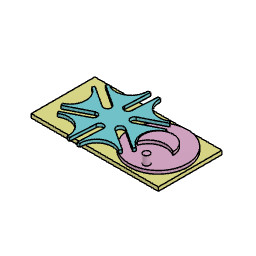
6 Slotted Geneva Mechanism v4 (Autodesk Fusion 360 design; units mm, degrees)
Autodesk Fusion 360 part; units mm, degrees
note: some values were not read from the file. Chosen so that the rebuilt part matches the saved one: which face or edge a step refers to. Set by a fixed rule: which sketch regions a step uses.
sketch "Holder" plane through (0, 0, 0) normal (0, 0, 1) x (1, 0, 0) in component "Holder"
  line L0 (100, -50) -> (-100, -50)
  line L1 (-100, -50) -> (-100, 50)
  line L2 (-100, 50) -> (100, 50)
  line L3 (100, 50) -> (100, -50)
  line L4 (100, -50) -> (-100, 50) construction
  line L5 (-100, -50) -> (100, 50) construction
  constraint horizontal L0
  constraint perpendicular L0 L1
  constraint parallel L0 L2
  constraint parallel L1 L3
  constraint coincident L4 origin
  constraint coincident L5 origin
extrude "Extrude1" add sketch "Holder" along normal blind 6 makes body 1 in component "Holder"
sketch "crank" plane through (0, 0, 6) normal (0, 0, 1) x (-1, 0, 0) in component "Crank"
  line L0 (-100, -50) -> (100, -50)
  line L1 (100, -50) -> (100, 50)
  line L2 (100, 50) -> (-100, 50)
  line L3 (-100, 50) -> (-100, -50)
  line L4 (100, 0) -> (-100, 0) construction
  line L5 (0, -50) -> (0, 50) construction
  line L6 (0, 0) -> (-100, 0) construction
  line L7 (-50, 0) -> (-50, -50) construction
  circle A0 centre (-50, 0) radius 46.0977
  constraint midpoint L1 L4.start
  constraint midpoint L3 L4.end
  constraint midpoint L0 L5.start
  constraint midpoint L2 L5.end
  constraint coincident L6.start origin
  constraint midpoint L6 L7.start
  constraint coincident L0 L7.end
  constraint perpendicular L0 L7
  constraint coincident L7.start A0.centre
extrude "Extrude1'" add sketch "crank" along normal blind 5 separate body contours A0 makes body 2 in component "Crank"
sketch "rotating point" plane through (0, 0, 6) normal (0, 0, -1) x (1, 0, 0) in component "Crank"
  circle A0 centre (50, 0) radius 46.0977
  circle A1 centre (50, 0) radius 5
  dimension "d7" = 10
  constraint concentric A0 A1
  measures "d7" diameter of A1
sketch "crank hole" plane through (0, 0, 0) normal (0, 0, -1) x (1, 0, 0) in component "Holder"
  line L0 (-100, -50) -> (100, -50)
  line L1 (100, -50) -> (100, 50)
  line L2 (100, 50) -> (-100, 50)
  line L3 (-100, 50) -> (-100, -50)
  circle A0 centre (50, 0) radius 5
  dimension "d8" = 10
  measures "d8" diameter of A0
extrude "Extrude2" cut sketch "crank hole" against normal blind 21 contours A0 bodies 1 in component "Holder"
extrude "Extrude2'" add sketch "rotating point" along normal blind 6 contours A1 bodies 2 in component "Crank"
move_face "OffsetFaces1" offset -0.5 1 faces at (54.9938, 0.2492, 2) on bodies 2 in component "Crank"
sketch "middle circle" plane through (0, 0, 11) normal (0, 0, 1) x (-1, 0, 0) in component "Crank"
  circle A0 centre (-50, 0) radius 46.0977
  circle A1 centre (-50, 0) radius 24.5
  circle A2 centre (-74.4998, -0.0916) radius 27.5
  dimension "d14" = 49
  dimension "d15" = 55
  constraint concentric A0 A1
  constraint coincident A1 A2.centre
  measures "d14" diameter of A1
  measures "d15" diameter of A2
extrude "Extrude3" add sketch "middle circle" along normal blind 5 contours A1 A2 picked at (-40.002, 2.3523) bodies 2 in component "Crank"
sketch "contact rod" plane through (0, 0, 11) normal (0, 0, 1) x (-1, 0, 0) in component "Crank"
  arc A0 (-58.9812, -22.7945) -> (-59.1513, 22.7267) centre (-74.4998, -0.0916) ccw
  arc A1 (-58.9812, -22.7945) -> (-59.1513, 22.7267) centre (-50, 0) ccw
  circle A2 centre (-50, 0) radius 46.0977
  line L0 (-50, 0) -> (-95, 0) construction
  line L1 (-95, 0) -> (-72.5, 0) construction
  circle A3 centre (-83.75, 0) radius 5
  dimension "d18" = 10
  constraint coincident A1.centre A2.centre
  constraint horizontal L0
  constraint midpoint L0 L1.end
  constraint midpoint L1 A3.centre
  measures "d18" diameter of A3
extrude "Extrude4" add sketch "contact rod" against normal blind 5 contours A3 bodies 2 in component "Crank"
sketch "star " plane through (0, 0, 6) normal (0, 0, 1) x (-1, 0, 0) in component "Rotating star"
  circle A0 centre (-50, 0) radius 5
  line L0 (-100, -50) -> (100, -50)
  line L1 (100, -50) -> (100, 50)
  line L2 (100, 50) -> (-100, 50)
  line L3 (-100, 50) -> (-100, -50)
  line L4 (0, 0) -> (2.6271, 0)
  line L5 (2.6271, 0) -> (100, 0) construction
  line L6 (0, 0) -> (51.3135, 0) construction
  circle A1 centre (20, 0) radius 63.198
  circle A2 centre (-50, 0) radius 25
  dimension "d21" = 50
  constraint coincident L4.start L6.start
  constraint horizontal L4
  constraint midpoint L1 L5.end
  constraint perpendicular L1 L5
  constraint midpoint L5 L6.end
  constraint coincident L5 A1.centre
  constraint concentric A0 A2
  measures "d21" diameter of A2
extrude "Extrude1''" add sketch "star " along normal blind 10 separate body contours L0 L2 A1 A2 | L0 A1 | L2 A1 makes body 3 in component "Rotating star"
move_face "OffsetFaces1'" offset -5 1 faces at (-28.1206, -36.1937, 6) on bodies 3 in component "Rotating star"
pattern_circular "C-Pattern1" count 6 over 360 about axis through (-20, 0, 16) along (0, 0, 1) of 2 faces at (38.0291, -21.9476, 14.3333) (27.6641, 11.2297, 14.3333) on bodies 3 in component "Rotating star"
sketch "Hole" plane through (0, 0, 16) normal (0, 0, 1) x (-1, 0, 0) in component "Rotating star"
  arc A0 (-29.0014, 39.9104) -> (9.9373, 62.3917) centre (-15, 60.6218) ccw
  arc A1 (-29.0014, 39.9104) -> (-39.0642, 22.4813) centre (20, 0) ccw
  arc A2 (-39.0642, -22.4813) -> (-39.0642, 22.4813) centre (-50, 0) ccw
  arc A3 (-39.0642, -22.4813) -> (-29.0014, -39.9104) centre (20, 0) ccw
  arc A4 (9.9373, -62.3917) -> (-29.0014, -39.9104) centre (-15, -60.6218) ccw
  arc A5 (9.9373, -62.3917) -> (30.0627, -62.3917) centre (20, 0) ccw
  arc A6 (69.0014, -39.9104) -> (30.0627, -62.3917) centre (55, -60.6218) ccw
  arc A7 (69.0014, -39.9104) -> (79.0642, -22.4813) centre (20, 0) ccw
  arc A8 (79.0642, 22.4813) -> (79.0642, -22.4813) centre (90, 0) ccw
  arc A9 (79.0642, 22.4813) -> (69.0014, 39.9104) centre (20, 0) ccw
  arc A10 (30.0627, 62.3917) -> (69.0014, 39.9104) centre (55, 60.6218) ccw
  arc A11 (30.0627, 62.3917) -> (9.9373, 62.3917) centre (20, 0) ccw
  line L0 (25, 0) -> (-34.731, -31.599) construction
  line L1 (-2.3358, -7.6734) -> (-37.5367, -26.2954)
  arc A12 (-37.5367, -26.2954) -> (-31.9253, -36.9026) centre (-34.731, -31.599) ccw
  line L2 (-31.9253, -36.9026) -> (3.2756, -18.2805)
  arc A13 (3.2756, -18.2805) -> (-2.3358, -7.6734) centre (0.4699, -12.977) ccw
  line L3 (0.4699, -12.977) -> (-34.731, -31.599) construction
  dimension "d27" = 12
  constraint midpoint A3 L0.end
  constraint tangent L1 A12
  constraint tangent A12 L2
  constraint parallel L1 L2
  constraint tangent L2 A13
  constraint tangent L1 A13
  constraint coincident L0.end A12.centre
  constraint parallel L0 L3
  measures "d27" distance of L1 L2
extrude "Extrude2''" cut sketch "Hole" against normal blind 20 contours A3 L1 L2 A13 bodies 3 in component "Rotating star"
pattern_circular "C-Pattern2" count 6 over 360 about axis through (-20, 0, 16) along (0, 0, 1) of "Extrude2''" in component "Rotating star"
sketch "support " plane through (0, 0, 11) normal (0, 0, -1) x (1, 0, 0) in component "Rotating star"
  line L0 (-2.1867, 15.5067) -> (31.4876, 36.6471)
  arc A0 (31.4876, 36.6471) -> (29.0014, 39.9104) centre (-20, 0) ccw
  arc A1 (-9.9373, 62.3917) -> (29.0014, 39.9104) centre (15, 60.6218) ccw
  arc A2 (-9.9373, 62.3917) -> (-13.9853, 62.9111) centre (-20, 0) ccw
  line L1 (-13.9853, 62.9111) -> (-12.5308, 23.6241)
  arc A3 (-24.5226, 23.1801) -> (-12.5308, 23.6241) centre (-18.5267, 23.4021) ccw
  line L2 (-24.5226, 23.1801) -> (-25.9936, 62.9131)
  arc A4 (-25.9936, 62.9131) -> (-30.0627, 62.3917) centre (-20, 0) ccw
  arc A5 (-69.0014, 39.9104) -> (-30.0627, 62.3917) centre (-55, 60.6218) ccw
  arc A6 (-69.0014, 39.9104) -> (-71.4752, 36.6645) centre (-20, 0) ccw
  line L3 (-71.4752, 36.6645) -> (-36.7244, 18.2805)
  arc A7 (-42.3358, 7.6734) -> (-36.7244, 18.2805) centre (-39.5301, 12.977) ccw
  line L4 (-42.3358, 7.6734) -> (-77.4811, 26.266)
  arc A8 (-77.4811, 26.266) -> (-79.0642, 22.4813) centre (-20, 0) ccw
  arc A9 (-79.0642, -22.4813) -> (-79.0642, 22.4813) centre (-90, 0) ccw
  arc A10 (-79.0642, -22.4813) -> (-77.49, -26.2466) centre (-20, 0) ccw
  line L5 (-77.49, -26.2466) -> (-44.1936, -5.3435)
  arc A11 (-37.8133, -15.5067) -> (-44.1936, -5.3435) centre (-41.0034, -10.4251) ccw
  line L6 (-37.8133, -15.5067) -> (-71.4876, -36.6471)
  arc A12 (-71.4876, -36.6471) -> (-69.0014, -39.9104) centre (-20, 0) ccw
  arc A13 (-30.0627, -62.3917) -> (-69.0014, -39.9104) centre (-55, -60.6218) ccw
  arc A14 (-30.0627, -62.3917) -> (-26.0147, -62.9111) centre (-20, 0) ccw
  line L7 (-26.0147, -62.9111) -> (-27.4692, -23.6241)
  arc A15 (-15.4774, -23.1801) -> (-27.4692, -23.6241) centre (-21.4733, -23.4021) ccw
  line L8 (-15.4774, -23.1801) -> (-14.0064, -62.9131)
  arc A16 (-14.0064, -62.9131) -> (-9.9373, -62.3917) centre (-20, 0) ccw
  arc A17 (29.0014, -39.9104) -> (-9.9373, -62.3917) centre (15, -60.6218) ccw
  arc A18 (29.0014, -39.9104) -> (31.4752, -36.6645) centre (-20, 0) ccw
  line L9 (31.4752, -36.6645) -> (-3.2756, -18.2805)
  arc A19 (2.3358, -7.6734) -> (-3.2756, -18.2805) centre (-0.4699, -12.977) ccw
  line L10 (2.3358, -7.6734) -> (37.4811, -26.266)
  arc A20 (37.4811, -26.266) -> (39.0642, -22.4813) centre (-20, 0) ccw
  arc A21 (39.0642, 22.4813) -> (39.0642, -22.4813) centre (50, 0) ccw
  arc A22 (39.0642, 22.4813) -> (37.49, 26.2466) centre (-20, 0) ccw
  line L11 (37.49, 26.2466) -> (4.1936, 5.3435)
  arc A23 (-2.1867, 15.5067) -> (4.1936, 5.3435) centre (1.0034, 10.4251) ccw
  circle A24 centre (-20, 0) radius 5
  dimension "d32" = 10
  constraint concentric A0 A24
  measures "d32" diameter of A24
sketch "star hole" plane through (0, 0, 0) normal (0, 0, -1) x (1, 0, 0) in component "Holder"
  circle A0 centre (50, 0) radius 5
  line L0 (-100, -50) -> (100, -50)
  line L1 (100, -50) -> (100, 50)
  line L2 (100, 50) -> (-100, 50)
  line L3 (-100, 50) -> (-100, -50)
  circle A1 centre (-20, 0) radius 5.5
  dimension "d33" = 11
  measures "d33" diameter of A1
extrude "Extrude3'" cut sketch "star hole" against normal blind 50 contours A1 bodies 1 in component "Holder"
extrude "Extrude3''" add sketch "support " along normal blind 11 contours A24 bodies 3 in component "Rotating star"
move_face "OffsetFaces2" offset -1 1 faces at (40.0739, -22.3992, 14.3333) on bodies 2 in component "Crank"
sketch "crank for the contact rod" plane through (67.101, 46.9846, 11) normal (0, 0, 1) x (0.34202, 0.939693, 0)
  arc A0 (-26.5, 0.0354) -> (-67.9116, -15.2127) centre (-41.5345, -22.991) ccw
  arc A1 (-26.5, 0.0354) -> (-67.9116, -15.2127) centre (-50, 0) ccw
  circle A2 centre (-50, 0) radius 46.0977
sketch "contact rod (2)" plane through (67.101, 46.9846, 11) normal (0, 0, 1) x (0.34202, 0.939693, 0)
  line L0 (-73.8686, 65.8531) -> (-50, 0) construction
  line L1 (-50, 0) -> (-27.4519, 26.7987) construction
  line L2 (-27.4519, 26.7987) -> (-73.8686, 65.8531) construction
  circle A0 centre (-27.4519, 26.7987) radius 5
  dimension "d50" = 30
  dimension "d51" = 60
  dimension "d52" = 10
  constraint coincident L1.end L2.start
  measures "d50" angle of L0 L2
  measures "d51" angle of L0 L1
  measures "d52" diameter of A0
extrude "Extrude5" add sketch "contact rod (2)" along normal blind 14 sketch seen with x (-0.422618, -0.906308, 0) y (0.906308, -0.422618, 0) z (0, 0, 1) at (71.1309, 45.3154, 0) bodies 2 in component "Crank"
component "Holder" placed x (1, 0, 0) y (0, 1, 0) z (0, 0, 1) at (0, 0, 0)
component "Crank" placed x (-0.422618, 0.906308, 0) y (-0.906308, -0.422618, 0) z (0, 0, 1) at (71.1309, -45.3154, 0)
component "Rotating star" placed x (0.999949, -0.010082, 0) y (0.010082, 0.999949, 0) z (0, 0, 1) at (-0.001, -0.2016, 0)
named bodies: "Holder", "crank", "Star"
